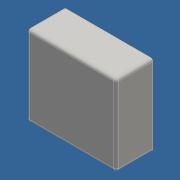
# Autodesk Inventor part: Board_cover
Saved by Autodesk Inventor 2016 (Build 200138000, 138)
## iProperties
Created: 2021-06-17
Part Number: Board_cover
Material: Generico
Document SubType Name: Modeling
Designer: Galli Davide
Density: 1 g/cm^3
Appearance: Default
Author: Galli Davide
Autodesk Inventor part; units mm, degrees
ref_plane "YZ Plane" through (0, 0, 0) normal (1, 0, 0) x (0, 1, 0)
ref_plane "XZ Plane" through (0, 0, 0) normal (0, 1, 0) x (-1, 0, 0)
ref_plane "XY Plane" through (0, 0, 0) normal (0, 0, 1) x (1, 0, 0)
sketch "Schizzo1" plane through (0, 0, 0) normal (0, 1, 0) x (-1, 0, 0)
  line L0 (0, 0) -> (71, 0)
  line L1 (71, 0) -> (71, -64)
  line L2 (71, -64) -> (0, -64)
  line L3 (0, -64) -> (0, 0)
  dimension "d0" = 71
  dimension "d1" = 64
  constraints: 8 end point, 2 parallel, 1 horizontal, 1 perpendicular
  measures "d0" distance of L1.end L2.end
  measures "d1" distance of L0.end L1.end
extrude "Estrusione1" add sketch "Schizzo1" along normal blind 29
shell "Svuotamento1" thickness 2 removed faces 1 at (-23.6667, 29, -21.3333)
fillet "Raccordo1" radius 2 4 edges at (0, 0, -32) (-35.5, 0, -64) (-35.5, 0, 0) (-71, 0, -32)
fillet "Raccordo2" radius 2 8 edges at (-0.5858, 0.5858, -63.4142) (0, 15.5, -64) (-0.5858, 0.5858, -0.5858) (0, 15.5, 0) (-70.4142, 0.5858, -63.4142) (-71, 15.5, -64) (-70.4142, 0.5858, -0.5858) (-71, 15.5, 0)
sketch "Schizzo3" plane through (-71, 2, -2) normal (-1, 0, 0) x (0, 0, 1)
  line L0 (-52.5, 27) -> (-27.5, 27)
  line L1 (-27.5, 27) -> (-27.5, 15)
  line L2 (-27.5, 15) -> (-52.5, 15)
  line L3 (-52.5, 15) -> (-52.5, 27)
  line L4 (-62, 27) -> (-62, 0) projected
  line L5 (-60, 27) -> (0, 27) projected
  line L6 (-60, 0) -> (-60, 27) projected
  line L7 (-60, 0) -> (-60, 27) projected
  point P0 (2, -2)
  dimension "d16" = 0
  dimension "d17" = 12
  dimension "d23" = 7.5
  dimension "d24" = 25
  constraints: 8 end point, 2 parallel, 1 horizontal, 1 perpendicular
  measures "d16" distance between parallel lines of L0 L5
  measures "d17" distance of L0.end L1.end
  measures "d23" distance between parallel lines of L3 L6
  measures "d24" distance of L1.end L2.end
extrude "Estrusione3" cut sketch "Schizzo3" against normal up to next
chamfer "Smusso2" distance 2 angle 45 4 edges at (-70, 29, -54.5) (-70, 29, -29.5) (-70, 17, -29.5) (-70, 17, -54.5)
